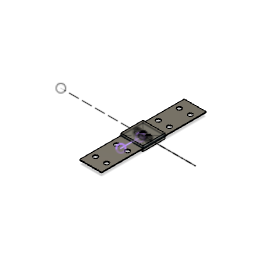
pretensioned sheet v2 (Autodesk Fusion 360 design; units mm, degrees)
Autodesk Fusion 360 part; units mm, degrees
note: some values were not read from the file. Set by a fixed rule: which face or edge a step refers to.
sketch "Sketch1" plane through (0, 0, 0) normal (0, 1, 0) x (1, 0, 0)
  line L0 (10, -10) -> (-10, -10)
  line L1 (-10, -10) -> (-10, 10)
  line L2 (-10, 10) -> (10, 10)
  line L3 (10, 10) -> (10, -10)
  line L4 (10, -10) -> (-10, 10) construction
  line L5 (-10, -10) -> (10, 10) construction
  line L6 (0, 0) -> (47.3692, 0) construction
  line L7 (47.3692, 0) -> (-74.5254, 0) construction
  circle A0 centre (5, 0) radius 2
  line L8 (0, -20) -> (0, -2.5)
  circle A1 centre (-5, 0) radius 2
  dimension "d1" = 20
  dimension "d2" = 20
  dimension "d3" = 4
  dimension "d4" = 5
  constraint horizontal L0
  constraint perpendicular L0 L1
  constraint parallel L0 L2
  constraint parallel L1 L3
  constraint coincident L4 L6.start
  constraint coincident L5 L6.start
  constraint coincident L6.start origin
  constraint parallel L0 L6
  constraint perpendicular L3 L7
  constraint coincident L6 A0.centre
  constraint symmetric A0 L8 A1
  measures "d1" distance of L1.end L2.end
  measures "d2" distance of L0.end L1.end
  measures "d3" diameter of A0
  measures "d4" distance of L6.start A0.centre
extrude "Extrude1" add sketch "Sketch1" along normal blind 2 contours L0 L1 L2 L3 | A0 | A1 makes body 1
extrude "Extrude2" add sketch "Sketch1" against normal blind 0.6 separate body makes body 2
extrude "Extrude3" add sketch "Sketch1" against normal blind 2 from surface at -0.6 separate body makes body 3
move_face "OffsetFaces1" offset -0.1 2 faces at (6.9901, -1.2667, 0.1991) (-3.0099, -1.2667, 0.1991) on bodies 3
chamfer "Chamfer1" distance 1 angle 45 2 edges at (3.0421, -2.6, 0.7594) (-6.9579, -2.6, 0.7594) on bodies 3
extrude "Extrude4" add sketch "Sketch1" against normal blind 3.6 contours A0 | A1 bodies 1
move_face "OffsetFaces2" offset -0.5 2 faces at (6.6667, -0.4, 10) (-3.3333, -0.2, -10) on bodies 2
pattern_linear "R-Pattern1" count 5 spacing 19 along (0, 0, 1) both ways of bodies 2 makes body 4 at (-1.4231, 0, -44.9539) makes body 5 at (-1.4231, 0, -25.9539) makes body 6 at (-1.4231, 0, 12.0461) makes body 7 at (-1.4231, 0, 31.0461)
combine "Combine1" operation add target body 2 tool bodies 7 6 5 4
named bodies: "pretensioned sheet tile", "pretensioned sheet sheet", "pretensioned sheet backer", "sheet (1)", "sheet (2)", "sheet (3)", "sheet (4)"
